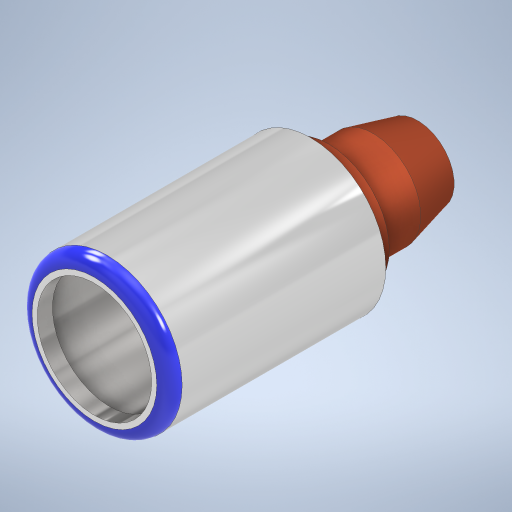
# Autodesk Inventor part: Колибри-Шаблон
Saved by Autodesk Inventor 2023 (Build 270158000, 158)
## iProperties
Created: 2024-01-28
Part Number: Колибри-Шаблон
Material: Типовые
Document SubType Name: Modeling
Designer: user
Density: 1 g/cm^3
Appearance: Рифленый 45
Author: user
Autodesk Inventor part; units mm, degrees
ref_plane "YZ Plane" through (0, 0, 0) normal (1, 0, 0) x (0, 1, 0)
ref_plane "XZ Plane" through (0, 0, 0) normal (0, 1, 0) x (-1, 0, 0)
ref_plane "XY Plane" through (0, 0, 0) normal (0, 0, 1) x (1, 0, 0)
sketch "Эскиз1" plane through (0, 0, 0) normal (0, 0, 1) x (1, 0, 0)
  circle A0 centre (0, 0) radius 59
  dimension "d0" = 118
  constraints: 1 centre point, 1 coincident
  measures "d0" diameter of A0
extrude "Выдавливание1" add sketch "Эскиз1" along normal blind 150
extrude "Выдавливание2" add sketch "Эскиз1" against normal blind 4 draft -70
sketch "Эскиз2" plane through (0, 0, -4) normal (0, 0, -1) x (-1, 0, 0)
  circle A0 centre (0, 0) radius 47.803848
  constraints: 1 centre point, 1 coincident
extrude "Выдавливание3" add sketch "Эскиз2" along normal blind 10
sketch "Эскиз3" plane through (0, 0, -14) normal (0, 0, -1) x (-1, 0, 0)
  circle A0 centre (0, 0) radius 37.5
  circle A1 centre (0, 0) radius 36.5
  dimension "d7" = 75
  dimension "d20" = 73
  constraints: 2 centre point, 2 coincident
  measures "d7" diameter of A0
  measures "d20" diameter of A1
extrude "Выдавливание4" add sketch "Эскиз3" along normal blind 35 contours A0 | A1
sketch "Эскиз4" plane through (0, 0, -49) normal (0, 0, -1) x (-1, 0, 0)
  point P0 (0, 0)
sketch "Эскиз5" plane through (0, 0, -49) normal (0, 0, -1) x (-1, 0, 0)
  circle A0 centre (0, 0) radius 37.5
  circle A1 centre (0, 0) radius 35
  dimension "d16" = 70
  constraints: 2 centre point, 2 coincident
  measures "d16" diameter of A1
sketch "Эскиз5 outline for Выдавливание5" plane through (0, 0, -49) normal (0, 0, -1) x (-1, 0, 0)
  circle A0 centre (0, 0) radius 37.5
extrude "Выдавливание5" add sketch "Эскиз5 outline for Выдавливание5" along normal blind 35 draft -14
sketch "Эскиз6" plane through (0, 0, 150) normal (0, 0, 1) x (1, 0, 0)
  circle A0 centre (0, 0) radius 59
  circle A1 centre (0, 0) radius 45
  dimension "d12" = 90
  constraints: 2 centre point, 2 coincident
  measures "d12" diameter of A1
extrude "Выдавливание6" add sketch "Эскиз6" along normal blind 20
fillet "Сопряжение1" radius 10 1 edges at (-59, 0, 170)
sketch "Эскиз7" plane through (0, 0, -84) normal (0, 0, -1) x (-1, 0, 0)
  circle A0 centre (0, 0) radius 28.77352
  circle A1 centre (0, 0) radius 27.5
  dimension "d17" = 55
  constraints: 2 centre point, 2 coincident
  measures "d17" diameter of A1
extrude "Выдавливание7" cut sketch "Эскиз7" against normal blind 35 draft 15 contours A1
sketch "Эскиз8" plane through (0, 0, -49) normal (0, 0, -1) x (-1, 0, 0)
  circle A0 centre (0, 0) radius 36.5
  dimension "d21" = 73
  constraints: 1 centre point, 1 coincident
  measures "d21" diameter of A0
extrude "Выдавливание8" cut sketch "Эскиз8" against normal blind 35
sketch "Эскиз9" plane through (0, 0, -14) normal (0, 0, -1) x (-1, 0, 0)
  circle A0 centre (0, 0) radius 36.5
  dimension "d24" = 73
  constraints: 1 centre point, 1 coincident
  measures "d24" diameter of A0
extrude "Выдавливание9" cut sketch "Эскиз9" against normal blind 10
sketch "Эскиз10" plane through (0, 0, -4) normal (0, 0, -1) x (-1, 0, 0)
  circle A0 centre (0, 0) radius 36.5
  dimension "d27" = 73
  constraints: 1 centre point, 1 coincident
  measures "d27" diameter of A0
extrude "Выдавливание10" cut sketch "Эскиз10" against normal blind 4 draft 78
sketch "Эскиз11" plane through (0, 0, 0) normal (0, 0, -1) x (-1, 0, 0)
  circle A0 centre (0, 0) radius 58
  dimension "d30" = 116
  constraints: 1 centre point, 1 coincident
  measures "d30" diameter of A0
extrude "Выдавливание11" cut sketch "Эскиз11" against normal blind 158
